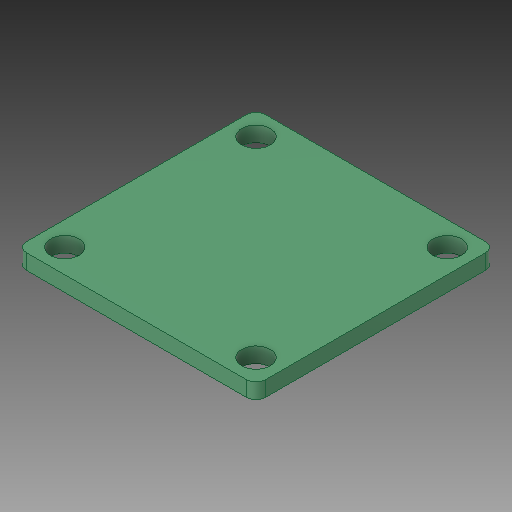
# Autodesk Inventor part: Large Encoder PCB
Saved by Autodesk Inventor 2018.2 (Build 222227000, 227)
## iProperties
Created: 2018-02-27
Part Number: Large Encoder PCB
Material: Generic
Document SubType Name: Modeling
Designer: Moochster
Density: 1 g/cm^3
Appearance: Smooth - Dark Sea Green
Mass: 0.953388 g
Surface Area: 14.0931 cm^2
Volume: 0.953388 cm^3
Author: Moochster
Autodesk Inventor part; units mm, degrees
ref_plane "YZ Plane" through (0, 0, 0) normal (1, 0, 0) x (0, 1, 0)
ref_plane "XZ Plane" through (0, 0, 0) normal (0, 1, 0) x (-1, 0, 0)
ref_plane "XY Plane" through (0, 0, 0) normal (0, 0, 1) x (1, 0, 0)
sketch "Sketch1" plane through (0, 0, 0) normal (0, 1, 0) x (-1, 0, 0)
  line L0 (0, 0) -> (-25, 0)
  line L1 (-25, 0) -> (-25, -25)
  line L2 (-25, -25) -> (0, -25)
  line L3 (0, -25) -> (0, 0)
  line L4 (-2.5, -22.5) -> (-22.5, -22.5) construction
  line L5 (-22.5, -22.5) -> (-22.5, -2.5) construction
  line L6 (-22.5, -2.5) -> (-2.5, -2.5) construction
  line L7 (-2.5, -2.5) -> (-2.5, -22.5) construction
  dimension "d0" = 25
  dimension "d1" = 25
  dimension "d2" = 20
  dimension "d3" = 20
  dimension "d4" = 2.5
  dimension "d5" = 2.5
  constraints: 16 end point, 4 coincident, 4 parallel, 2 horizontal, 2 perpendicular
  measures "d0" distance of L2.end L1.end
  measures "d1" distance of L1.end L0.end
  measures "d2" distance of L4.end L5.end
  measures "d3" distance of L4.start L4.end
  measures "d4" distance between parallel lines of L2 L4
  measures "d5" distance between parallel lines of L3 L7
extrude "Extrusion1" add sketch "Sketch1" along normal blind 1.6
hole "Hole1" at (2.5, 0, -22.5) at (2.5, 0, -2.5) at (22.5, 0, -2.5) at (22.5, 0, -22.5) direction (0, 1, 0) diameter 3 depth 8 tip angle 118
fillet "Fillet1" radius 1 4 edges at (25, 0.8, -25) (25, 0.8, 0) (0, 0.8, -25) (0, 0.8, 0)
body "Solid1"
